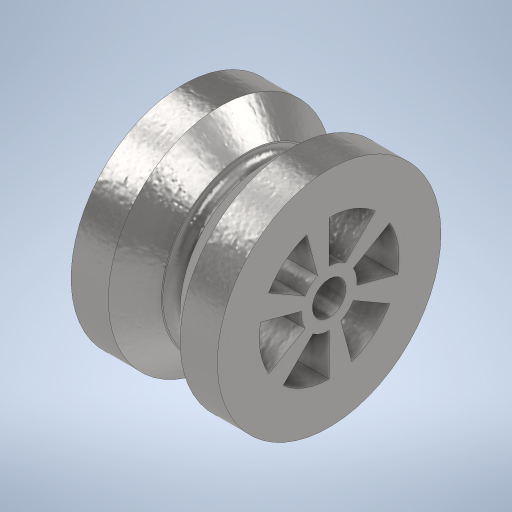
# Autodesk Inventor part: Rad
Saved by Autodesk Inventor 2024 (Build 280153000, 153)
## iProperties
Created: 2024-02-12
Part Number: Rad
Material: Stahl, galvanisiert
Document SubType Name: Modeling
Designer: ffogue
Density: 7.85 g/cm^3
Appearance: Galvanisiert
Author: ffogue
Autodesk Inventor part; units mm, degrees
ref_plane "YZ Plane" through (0, 0, 0) normal (1, 0, 0) x (0, 1, 0)
ref_plane "XZ Plane" through (0, 0, 0) normal (0, 1, 0) x (-1, 0, 0)
ref_plane "XY Plane" through (0, 0, 0) normal (0, 0, 1) x (1, 0, 0)
sketch "Skizze1" plane through (0, 0, 0) normal (0, 0, 1) x (1, 0, 0)
  line L0 (0, 0) -> (7.85, 0)
  line L1 (3.925, 0) -> (3.925, 15.4029) construction
  line L2 (0, 0) -> (0, 6)
  line L3 (0, 6) -> (2, 6)
  line L4 (2, 6) -> (3.425, 4.575)
  line L5 (3.425, 4.575) -> (3.425, 4.5)
  arc A0 (3.425, 4.5) -> (4.425, 4.5) centre (3.925, 4.5) ccw
  line L6 (4.425, 4.5) -> (4.425, 4.575)
  line L7 (4.425, 4.575) -> (5.85, 6)
  line L8 (5.85, 6) -> (7.85, 6)
  line L9 (7.85, 6) -> (7.85, 0)
  dimension "d0" = 2
  dimension "d1" = 45
  dimension "d2" = 0.5
  dimension "d3" = 12
  dimension "d4" = 9
  dimension "d5" = 7.85
  constraints: 20 end point, 3 equal length, 2 parallel, 2 perpendicular, 2 point on circle, 2 point on line, 2 tangent, 2 vertical, 1 centre point, 1 coincident, 1 horizontal, 1 horizontal alignment, 1 midpoint, 1 symmetric about line
  measures "d0" distance of L2.end L3.end
  measures "d1" angle of L3 L4
  measures "d2" radius of A0
  measures "d3" diameter of L3 L0
  measures "d4" diameter of A0.centre L0
  measures "d5" distance of L0.start L0.end
revolve "Umdrehung1" add sketch "Skizze1" angle 360 about axis through (0, 0, 0) along (1, 0, 0)
sketch "Skizze2" plane through (7.85, 0, 0) normal (1, 0, 0) x (0, 0, -1)
  circle A0 centre (0, 0) radius 6 projected
  circle A1 centre (0, 0) radius 1.5
  line L0 (-0.869, 1.2226) -> (-2.469, 2.8225)
  line L1 (-1.2226, 0.869) -> (-2.8225, 2.469)
  line L2 (8.4, 0) -> (-8.4, 0) projected
  line L3 (0, 0) -> (-2.6517, 2.6517) construction
  circle A2 centre (0, 0) radius 3.75
  line L4 (-1.5, 0) -> (-3.75, 0)
  dimension "d7" = 3
  dimension "d8" = 45
  dimension "d9" = 0.5
  dimension "d10" = 7.5
  constraints: 8 end point, 7 point on circle, 2 centre point, 2 coincident, 2 parallel, 2 point on line, 1 other
  measures "d7" diameter of A1
  measures "d8" angle of L2 L0
  measures "d9" distance between parallel lines of L1 L0
  measures "d10" diameter of A2
extrude "Extrusion2" cut sketch "Skizze2" against normal through all contours A2 L1 A1 L2
pattern_circular "Runde Anordnung2" count 6 over 360 about axis through (6.85, 0, 0) along (1, 0, 0) of "Extrusion2"
sketch "Skizze3" plane through (7.85, 0, 0) normal (1, 0, 0) x (0, 0, -1)
  circle A0 centre (0, 0) radius 0.9
  dimension "d21" = 1.8
  constraints: 1 centre point, 1 coincident
  measures "d21" diameter of A0
extrude "Extrusion3" cut sketch "Skizze3" against normal up to surface (7.85 mm away)
